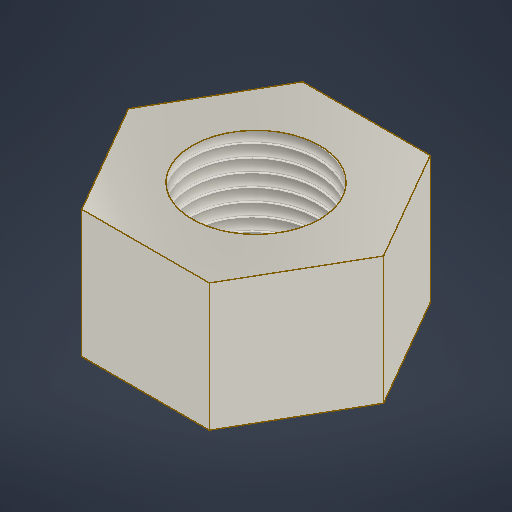
# Autodesk Inventor part: NutA
Saved by Autodesk Inventor 2026 (Build 300175000, 175)
## iProperties
Created: 2025-11-04
Part Number: NutA
Material: Titanium
Document SubType Name: Modeling
Designer: Study
Density: 4.51 g/cm^3
Appearance: Titanium
Mass: 8.17518 g
Surface Area: 12.7669 cm^2
Volume: 1.81268 cm^3
Author: Study
Autodesk Inventor part; units mm, degrees
ref_plane "YZ Plane" through (0, 0, 0) normal (1, 0, 0) x (0, 1, 0)
ref_plane "XZ Plane" through (0, 0, 0) normal (0, 1, 0) x (-1, 0, 0)
ref_plane "XY Plane" through (0, 0, 0) normal (0, 0, 1) x (1, 0, 0)
sketch "Sketch1" plane through (0, 0, 0) normal (0, 1, 0) x (-1, 0, 0)
  circle A0 centre (0, 0) radius 10 construction
  line L0 (10, 0) -> (5, -8.6603)
  line L1 (5, -8.6603) -> (-5, -8.6603)
  line L2 (-5, -8.6603) -> (-10, 0)
  line L3 (-10, 0) -> (-5, 8.6603)
  line L4 (-5, 8.6603) -> (5, 8.6603)
  line L5 (5, 8.6603) -> (10, 0)
  circle A1 centre (0, 0) radius 5
  dimension "d0" = 20
  dimension "d3" = 10
  constraints: 12 end point, 3 coincident, 1 centre point, 1 horizontal alignment, 15 other
  measures "d3" diameter of A1
extrude "Extrusion1" add sketch "Sketch1" along normal blind 10 contours L0 L1 L2 L3 L4 L5 | A1
extrude "Extrusion2" cut sketch "Sketch1" along normal blind 10 contours A1
thread "Thread1" size "M10x1" class "6H" standard "ISO Metric profile" length 10
body "Solid1"
